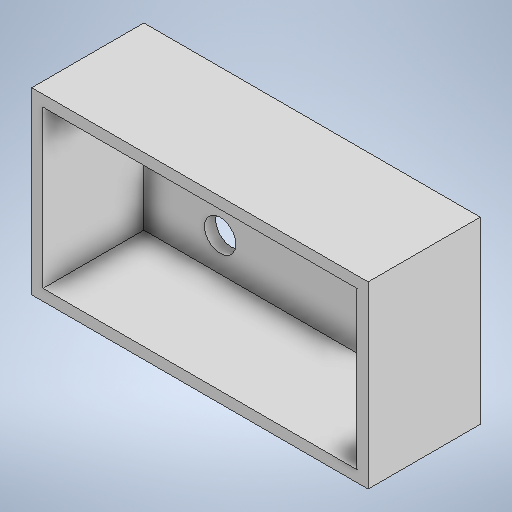
# Autodesk Inventor part: 제어부 커버
Saved by Autodesk Inventor 2025 (Build 290162000, 162)
## iProperties
Created: 2024-06-19
Part Number: 제어부 커버
Material: 일반
Document SubType Name: Modeling
Designer: goomi
Density: 1 g/cm^3
Appearance: 기본값
Author: goomi
Autodesk Inventor part; units mm, degrees
ref_plane "YZ Plane" through (0, 0, 0) normal (1, 0, 0) x (0, 1, 0)
ref_plane "XZ Plane" through (0, 0, 0) normal (0, 1, 0) x (-1, 0, 0)
ref_plane "XY Plane" through (0, 0, 0) normal (0, 0, 1) x (1, 0, 0)
sketch "스케치1" plane through (0, 0, 0) normal (0, 0, 1) x (1, 0, 0)
  line L0 (0, 0) -> (150, 0)
  line L1 (150, 0) -> (150, 80)
  line L2 (150, 80) -> (0, 80)
  line L3 (0, 80) -> (0, 0)
  line L4 (75, 80) -> (75, 65) construction
  line L5 (39, 90) -> (111, 90) construction
  line L6 (111, 90) -> (111, 40) construction
  line L7 (111, 40) -> (39, 40)
  line L8 (39, 40) -> (39, 90) construction
  line L9 (39, 90) -> (111, 40) construction
  line L10 (111, 90) -> (39, 40) construction
  line L11 (39, 40) -> (111, 40) construction
  line L12 (111, 40) -> (111, 65)
  line L13 (111, 65) -> (39, 65)
  line L14 (39, 65) -> (39, 40)
  line L15 (39, 40) -> (39, 20) construction
  line L16 (39, 20) -> (111, 20) construction
  circle A0 centre (39, 20) radius 7
  circle A1 centre (111, 20) radius 7
  line L17 (5, 75) -> (145, 75)
  line L18 (145, 75) -> (145, 5)
  line L19 (145, 5) -> (5, 5)
  line L20 (5, 5) -> (5, 75)
  dimension "d0" = 150
  dimension "d1" = 80
  dimension "d2" = 15
  dimension "d3" = 72
  dimension "d4" = 50
  dimension "d5" = 20
  dimension "d6" = 14
  dimension "d7" = 14
  dimension "d8" = 5
  constraints: 42 end point, 8 parallel, 5 perpendicular, 4 midpoint, 3 horizontal, 2 centre point, 2 coincident, 2 vertical, 3 other
  measures "d0" distance of L2.end L1.end
  measures "d1" distance of L1.end L0.end
  measures "d2" distance of L4.start L4.end
  measures "d3" distance of L6.end L7.end
  measures "d4" distance of L5.end L6.end
  measures "d5" distance of L7.end L15.end
  measures "d6" diameter of A0
  measures "d7" diameter of A1
  measures "d8" distance between parallel lines of L2 L17
extrude "돌출1" add sketch "스케치1" along normal blind 5 contours L17 L18 L19 L20
extrude "돌출2" add sketch "스케치1" along normal blind 50 contours L3 L2 L1 L0
